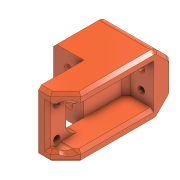
# Autodesk Inventor part: Print_Parts_A4
Saved by Autodesk Inventor 2020.1 (Build 241239000, 239)
## iProperties
Created: 2020-10-05
Part Number: Print_Parts_A4
Material: PC/ABS プラスチック
Document SubType Name: Modeling
Designer: kenta iguchi
Density: 0.357273 g/cm^3
Appearance: 滑らか - 淡いオレンジ
Author: kenta iguchi
Autodesk Inventor part; units mm, degrees
ref_plane "YZ Plane" through (0, 0, 0) normal (1, 0, 0) x (0, 1, 0)
ref_plane "XZ Plane" through (0, 0, 0) normal (0, 1, 0) x (-1, 0, 0)
ref_plane "XY Plane" through (0, 0, 0) normal (0, 0, 1) x (1, 0, 0)
sketch "スケッチ1" plane through (0, 0, 0) normal (0, 0, 1) x (1, 0, 0)
  line L0 (-10, -20) -> (10, -20)
  line L1 (10, -20) -> (10, 20)
  line L2 (10, 20) -> (-10, 20)
  line L3 (-10, 20) -> (-10, -20)
  line L4 (-10, -20) -> (10, 20) construction
  line L5 (10, -20) -> (-10, 20) construction
  point P0 (0, 0)
  dimension "d0" = 20
  dimension "d1" = 40
  constraints: 12 end point, 2 midpoint, 2 parallel, 1 horizontal, 1 perpendicular
  measures "d0" distance of L2.end L1.end
  measures "d1" distance of L1.end L0.end
extrude "押し出し1" add sketch "スケッチ1" along normal blind 40
sketch "Sketch6" plane through (10, -20, 0) normal (1, 0, 0) x (0, 0, -1)
  line L0 (0, 0) -> (0, 40) projected
  line L1 (0, 40) -> (-12, 40)
  line L2 (-12, 40) -> (-12, 0)
  line L3 (-12, 0) -> (0, 0)
  line L4 (0, 0) -> (0, 40)
  point P0 (0, 20)
  dimension "d33" = 12
  constraints: 8 end point, 2 parallel, 1 horizontal, 1 perpendicular
  measures "d33" distance between parallel lines of L0 L2
extrude "Extrusion4" add sketch "Sketch6" along normal blind 18
sketch "Sketch7" plane through (-10, -20, 40) normal (0, -1, 0) x (1, 0, 0)
  line L0 (20, -28) -> (20, 0) projected
  line L1 (20, -28) -> (38, -28) projected
  line L2 (20, 0) -> (38, 0)
  line L3 (38, 0) -> (38, -28)
  line L4 (38, -28) -> (20, -28)
  line L5 (20, -28) -> (20, 0)
  point P0 (10, -40)
  constraints: 8 end point, 2 parallel, 1 horizontal, 1 perpendicular
extrude "Extrusion5" add sketch "Sketch7" against normal blind 7.2
sketch "Sketch8" plane through (-10, 20, 40) normal (0, 1, 0) x (1, 0, 0)
  line L0 (38, 0) -> (38, 28) projected
  line L1 (20, 28) -> (38, 28) projected
  line L2 (20, 0) -> (20, 28) projected
  line L3 (20, 0) -> (38, 0) projected
  point P0 (10, 40)
extrude "Extrusion6" add sketch "Sketch8" against normal blind 7.2
chamfer "Chamfer3" distance 10 angle 45 2 edges at (9, -20, 0) (9, 20, 0)
sketch "Sketch9" plane through (0, 0, 0) normal (0, 0, -1) x (-1, 0, 0)
  line L0 (-28, 12.8) -> (-10, 12.8) projected
  line L1 (-10, -12.8) -> (-10, 12.8) projected
  line L2 (-10, -12.8) -> (-28, -12.8) projected
  line L3 (-28, 12.8) -> (-28, -12.8) projected
  point P0 (0, 0)
  point P1 (-20, -6)
  point P2 (-20, 6)
  dimension "d40" = 12
  dimension "d41" = 6
  dimension "d42" = 8
  constraints: 1 vertical alignment
  measures "d40" distance of point (-20, -6) point (-20, 6)
  measures "d41" vertical distance of point (-20, -6) point (0, 0)
  measures "d42" distance from line of L3 point (-20, -6)
hole "Hole3" at (20, 6, 0) at (20, -6, 0) direction (0, 0, 1) diameter 4.3 depth 58 counterbore diameter 6 counterbore depth 5
chamfer "Chamfer2" distance 3 angle 45 1 edges at (10, 0, 12)
sketch "Sketch10" plane through (0, 0, 0) normal (0, 0, -1) x (-1, 0, 0)
  circle A0 centre (-20, 6) radius 3 projected
  line L0 (-28, 10) -> (10, 10) projected
  line L1 (-28, -10) -> (-28, 10) projected
  line L2 (10, -10) -> (-28, -10) projected
  circle A1 centre (-20, -6) radius 3 projected
  line L3 (10, 10) -> (10, -10) projected
  line L4 (-28, 10) -> (10, 10) projected
  point P0 (0, 0)
  point P1 (-18.5639, 10)
  point P2 (0, -10)
  point P3 (0, 10)
  constraints: 2 vertical alignment, 1 point on line
hole "Hole4" at (0, -10, 0) at (0, 10, 0) direction (0, 0, 1) diameter 5.3 depth 58 counterbore diameter 9.5 counterbore depth 8
fillet "Fillet1" radius 5 6 edges at (9, -20, 10) (16.375, -10, 0) (-7.375, -10, 0) (-7.375, 10, 0) (16.375, 10, 0) (9, 20, 10)
chamfer "Chamfer6" distance 2 angle 45 8 edges at (-10, 20, 26.0355) (-10, 19.6194, 10.1577) (-10, 15, 5) (-10, 0, 0) (-10, -9.8423, 0.3806) (-10, -15, 5) (-10, -19.6194, 10.1577) (-10, -20, 26.0355)
sketch "Sketch15" plane through (0, 0, 40) normal (0, 0, 1) x (1, 0, 0)
  circle A0 centre (0, 10) radius 2.65 projected
  circle A1 centre (0, -10) radius 2.65 projected
  line L0 (-8, -20) -> (-10, -18) projected
  line L1 (-8, -20) -> (28, -20) projected
  line L2 (28, -20) -> (28, -12.8) projected
  line L3 (10, -12.8) -> (28, -12.8) projected
  line L4 (10, -12.8) -> (10, 12.8) projected
  line L5 (28, 12.8) -> (10, 12.8) projected
  line L6 (28, 20) -> (28, 12.8) projected
  line L7 (-8, 20) -> (28, 20) projected
  line L8 (-10, 18) -> (-8, 20) projected
  line L9 (-10, 18) -> (-10, -18) projected
  line L10 (-8, 20) -> (28, 20) projected
  line L11 (28, -20) -> (10, -20)
  line L12 (10, -20) -> (10, 20)
  line L13 (10, 20) -> (28, 20)
  line L14 (28, 20) -> (28, -20)
  point P0 (0, 0)
  point P1 (10, 20)
  constraints: 8 end point, 2 parallel, 1 horizontal, 1 midpoint, 1 perpendicular, 1 vertical alignment
extrude "Extrusion9" add sketch "Sketch15" along normal blind 30 contours L12 L3 L2 L1 | L12 L7 L6 L5
sketch "スケッチ16" plane through (0, 0, 70) normal (0, 0, 1) x (1, 0, 0)
  line L0 (28, -12.8) -> (10, -12.8) projected
  line L1 (13, -12.8) -> (13, 12.8) projected
  line L2 (13, -12.8) -> (28, -12.8) projected
  line L3 (28, 12.8) -> (28, -12.8) projected
  line L4 (28, 12.8) -> (13, 12.8) projected
  circle A0 centre (20, -6) radius 2.15 projected
  circle A1 centre (20, 6) radius 2.15 projected
  line L5 (28, 12.8) -> (28, 20) projected
  line L6 (28, 20) -> (10, 20) projected
  line L7 (10, 20) -> (10, 12.8) projected
  line L8 (10, 12.8) -> (28, 12.8) projected
  line L9 (10, 12.8) -> (13, 12.8) projected
  line L10 (10, 12.8) -> (10, -12.8) projected
  line L11 (13, -12.8) -> (10, -12.8) projected
  line L12 (13, -12.8) -> (13, 12.8) projected
  line L13 (13, -12.8) -> (28, -12.8) projected
  line L14 (10, 12.8) -> (16, 12.8)
  line L15 (16, 12.8) -> (16, -12.8)
  line L16 (16, -12.8) -> (10, -12.8)
  line L17 (10, -12.8) -> (10, 12.8)
  point P0 (0, 0)
  dimension "d98" = 6
  constraints: 8 end point, 2 parallel, 1 horizontal, 1 perpendicular, 1 point on line
  measures "d98" distance between parallel lines of L10 L15
extrude "押し出し10" add sketch "スケッチ16" against normal blind 12 contours L0 L1 L4 L15 | L0 L10 L8 L1
chamfer "面取り13" distance 5 angle 45 2 edges at (13, -12.8, 58) (13, 12.8, 58)
sketch "スケッチ17" plane through (16, -12.8, 70) normal (1, 0, 0) x (0, 0, -1)
  line L0 (0, 0) -> (0, 25.6) projected
  arc A0 (61.4645, 31.3355) -> (57.9289, 32.8) centre (57.9289, 27.8) ccw projected
  line L1 (57.9289, 32.8) -> (0, 32.8) projected
  line L2 (0, 25.6) -> (0, 32.8) projected
  line L3 (58, 25.6) -> (0, 25.6) projected
  line L4 (58, 25.6) -> (58, 0) projected
  line L5 (58, 0) -> (0, 0) projected
  line L6 (0, -7.2) -> (0, 0) projected
  line L7 (57.9289, -7.2) -> (0, -7.2) projected
  arc A1 (57.9289, -7.2) -> (61.4645, -5.7355) centre (57.9289, -2.2) ccw projected
  line L8 (68.5355, 1.3355) -> (61.4645, -5.7355) projected
  line L9 (70, 4.8711) -> (70, 20.7289) projected
  line L10 (61.4645, 31.3355) -> (68.5355, 24.2645) projected
  arc A2 (70, 20.7289) -> (68.5355, 24.2645) centre (65, 20.7289) ccw projected
  arc A3 (68.5355, 1.3355) -> (70, 4.8711) centre (65, 4.8711) ccw projected
  point P0 (70, 12.8)
  point P1 (6, 2.8)
  point P2 (6, 22.8)
  dimension "d104" = 10
  dimension "d105" = 10
  dimension "d106" = 6
  constraints: 1 vertical alignment
  measures "d104" distance from line of point (6, 22.8) L1
  measures "d105" distance from line of point (6, 2.8) L7
  measures "d106" distance from line of point (6, 2.8) L0
hole "穴5" at (16, -10, 64) at (16, 10, 64) direction (-1, 0, 0) diameter 4.3 depth 10
sketch "スケッチ18" plane through (16, -12.8, 70) normal (1, 0, 0) x (0, 0, -1)
  circle A0 centre (6, 2.8) radius 2.15 projected
  circle A1 centre (6, 22.8) radius 2.15 projected
  point P0 (70, 12.8)
hole "穴6" at (16, -10, 64) at (16, 10, 64) direction (1, 0, 0) diameter 8 end through all
fillet "フィレット3" radius 5 4 edges at (13, -12.8, 53) (13, -7.8, 58) (13, 12.8, 53) (13, 7.8, 58)
chamfer "Chamfer11" distance 10 angle 45 2 edges at (28, -16.4, 70) (28, 16.4, 70)
chamfer "面取り14" distance 2 angle 45 23 edges at (28, 20, 36.0355) (28, 19.6194, 10.1577) (28, 15, 5) (28, 0, 0) (28, -9.8423, 0.3806) (28, -15, 5) (28, -19.6194, 10.1577) (28, -20, 36.0355) (23, 20, 65) (14, 20, 70) (23, -20, 65) (14, -20, 70) (24, -14, 64) (19.5717, -12.8, 68.4283) (28, -12.8, 36) (27.4283, -12.8, 60.5717) (28, 12.8, 36) (24, 14, 64) (19.5717, 12.8, 68.4283) (17, 12.8, 70) (17, -12.8, 70) (16, 0, 70) (27.4283, 12.8, 60.5717)
sketch "スケッチ19" plane through (20, -6, 5) normal (0, 0, -1) x (-1, 0, 0)
  circle A0 centre (0, 0) radius 3 projected
  circle A1 centre (0, 12) radius 2.15 projected
  point P0 (20, 6)
hole "穴7" at (20, -6, 5) at (20, 6, 5) direction (0, 0, -1) diameter 8 depth 58
equation "\"d41\" = 0.5 * d40"
